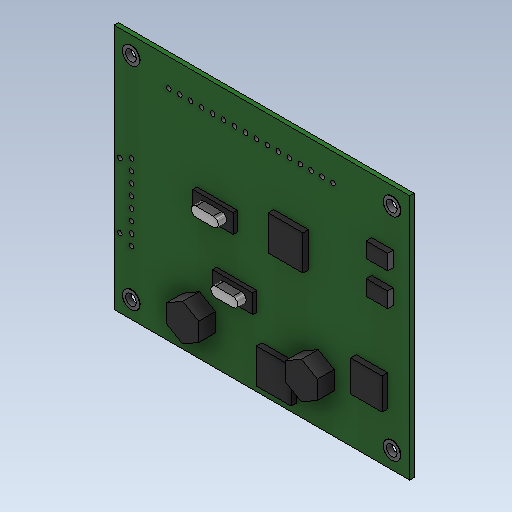
# Autodesk Inventor part: CPU_PCB
Saved by Autodesk Inventor 2020.1 (Build 241239000, 239)
## iProperties
Created: 2005-03-02
Part Number: CPU_PCB
Document SubType Name: Modeling
Designer: Autodesk
Density: 1 g/cm^3
Mass: 20.0863 g
Surface Area: 248.892 cm^2
Volume: 20.0863 cm^3
Material: Generic
Appearance: Default
Total Footprint: 0.000 kg
Author: Autodesk
Autodesk Inventor part; units mm, degrees
ref_plane "YZ Plane" through (0, 0, 0) normal (1, 0, 0) x (0, 1, 0)
ref_plane "XZ Plane" through (0, 0, 0) normal (0, 1, 0) x (-1, 0, 0)
ref_plane "XY Plane" through (0, 0, 0) normal (0, 0, 1) x (1, 0, 0)
sketch "Sketch1" plane through (0, 0, 0) normal (0, 0, 1) x (1, 0, 0)
  line L0 (-6.35, -62.4) -> (101.65, -62.4)
  line L1 (101.65, -62.4) -> (101.65, -152.4)
  line L2 (101.65, -152.4) -> (-6.35, -152.4)
  line L3 (-6.35, -152.4) -> (-6.35, -62.4)
  line L4 (0, -68.75) -> (95.3, -68.75) construction
  line L5 (95.3, -68.75) -> (95.3, -146.05) construction
  line L6 (95.3, -146.05) -> (0, -146.05) construction
  line L7 (0, -146.05) -> (0, -68.75) construction
  circle A0 centre (0, -146.05) radius 1.9812
  circle A1 centre (95.3, -146.05) radius 1.9812
  circle A2 centre (95.3, -68.75) radius 1.9812
  circle A3 centre (0, -68.75) radius 1.9812
  point P0 (47.65, -152.4)
  point P1 (47.65, -146.05)
  point P2 (-6.35, -107.4)
  point P3 (0, -107.4)
  dimension "d0" = 6.35
  dimension "d1" = 6.35
  dimension "d2" = 3.9624
  dimension "d84" = 90
  dimension "d85" = 108
  constraints: 16 end point, 4 centre point, 4 coincident, 4 midpoint, 4 parallel, 3 equal radius, 2 horizontal, 2 perpendicular, 1 horizontal alignment, 1 vertical alignment, 1 other
  measures "d0" distance between parallel lines of L3 L7
  measures "d1" distance between parallel lines of L0 L4
  measures "d2" diameter of A0
  measures "d84" distance between parallel lines of L2 L0
  measures "d85" distance between parallel lines of L3 L1
extrude "Extrusion1" add sketch "Sketch1" along normal blind 1.5875
sketch "Sketch2" plane through (0, 0, 1.5875) normal (0, 0, 1) x (1, 0, 0)
  circle A0 centre (0, -68.75) radius 1.9812 projected
  circle A1 centre (95.3, -68.75) radius 1.9812 projected
  circle A2 centre (95.3, -146.05) radius 1.9812 projected
  circle A3 centre (0, -146.05) radius 1.9812 projected
  line L0 (101.65, -62.4) -> (101.65, -152.4) projected
  line L1 (-6.35, -62.4) -> (101.65, -62.4) projected
  line L2 (-6.35, -152.4) -> (-6.35, -62.4) projected
  line L3 (101.65, -152.4) -> (-6.35, -152.4) projected
  circle A4 centre (0, -68.75) radius 3.175
  circle A5 centre (95.3, -68.75) radius 3.175
  circle A6 centre (95.3, -146.05) radius 3.175
  circle A7 centre (0, -146.05) radius 3.175
  dimension "d5" = 6.35
  constraints: 4 centre point, 4 coincident, 3 equal radius
  measures "d5" diameter of A7
extrude "Extrusion2" add sketch "Sketch2" along normal blind 0.1984 contours A4 | A5 | A6 | A7
sketch "Sketch3" plane through (0, 0, 0) normal (0, 0, -1) x (-1, 0, 0)
  circle A0 centre (0, -68.75) radius 1.9812 projected
  circle A1 centre (-95.3, -68.75) radius 1.9812 projected
  circle A2 centre (-95.3, -146.05) radius 1.9812 projected
  circle A3 centre (0, -146.05) radius 1.9812 projected
  line L0 (6.35, -62.4) -> (-101.65, -62.4) projected
  line L1 (-101.65, -62.4) -> (-101.65, -152.4) projected
  line L2 (-101.65, -152.4) -> (6.35, -152.4) projected
  line L3 (6.35, -152.4) -> (6.35, -62.4) projected
  circle A4 centre (0, -68.75) radius 3.175
  circle A5 centre (-95.3, -68.75) radius 3.175
  circle A6 centre (-95.3, -146.05) radius 3.175
  circle A7 centre (0, -146.05) radius 3.175
  dimension "d8" = 6.35
  constraints: 4 centre point, 4 coincident, 3 equal radius
  measures "d8" diameter of A4
extrude "Extrusion3" add sketch "Sketch3" along normal blind 0.1984 contours A4 | A5 | A6 | A7
sketch "Sketch4" plane through (0, 0, 1.5875) normal (0, 0, 1) x (1, 0, 0)
  circle A0 centre (95.3, -146.05) radius 3.175 projected
  circle A1 centre (0, -68.75) radius 3.175 projected
  circle A2 centre (95.3, -68.75) radius 3.175 projected
  circle A3 centre (0, -146.05) radius 3.175 projected
  line L0 (101.65, -62.4) -> (101.65, -152.4) projected
  line L1 (-6.35, -62.4) -> (101.65, -62.4) projected
  line L2 (-6.35, -152.4) -> (-6.35, -62.4) projected
  line L3 (101.65, -152.4) -> (-6.35, -152.4) projected
  circle A4 centre (0, -101.4) radius 1.6433
  circle A5 centre (0, -105.3624) radius 1.6433
  circle A6 centre (0, -109.3248) radius 1.6433
  circle A7 centre (0, -113.2872) radius 1.6433
  circle A8 centre (0, -117.2496) radius 1.6433
  circle A9 centre (0, -121.212) radius 1.6433
  circle A10 centre (0, -125.1744) radius 1.6433
  circle A11 centre (0, -129.1368) radius 1.6433
  circle A12 centre (-4.2418, -103.3812) radius 1.6433
  circle A13 centre (-4.2418, -127.1556) radius 1.6433
  line L4 (-6.35, -62.4) -> (101.65, -62.4) projected
  point P0 (13.65, -72.4)
  point P1 (17.65, -72.4)
  point P2 (21.65, -72.4)
  point P3 (25.65, -72.4)
  point P4 (29.65, -72.4)
  point P5 (33.65, -72.4)
  point P6 (37.65, -72.4)
  point P7 (41.65, -72.4)
  point P8 (45.65, -72.4)
  point P9 (49.65, -72.4)
  point P10 (53.65, -72.4)
  point P11 (57.65, -72.4)
  point P12 (61.65, -72.4)
  point P13 (65.65, -72.4)
  point P14 (69.65, -72.4)
  point P15 (73.65, -72.4)
  dimension "d22" = 3.9624
  dimension "d27" = 4.2418
  dimension "d28" = 1.9812
  dimension "d29" = 1.9812
  dimension "d30" = 4.2418
  dimension "d75" = 6.35
  dimension "d76" = 51
  dimension "d79" = 4
  dimension "d86" = 10
  dimension "d87" = 20
  constraints: 10 centre point, 2 equal radius, 1 horizontal, 1 vertical, 29 other
  measures "d22" distance of A4.centre A5.centre
  measures "d27" horizontal distance of A4.centre A12.centre
  measures "d28" vertical distance of A12.centre A4.centre
  measures "d29" vertical distance of A13.centre A11.centre
  measures "d30" horizontal distance of A13.centre A11.centre
  measures "d75" distance from line of L2 A4.centre
  measures "d76" distance from line of A4.centre L3
  measures "d79" distance of point (13.65, -72.4) point (17.65, -72.4)
  measures "d86" distance from line of L1 point (13.65, -72.4)
  measures "d87" distance from line of L2 point (13.65, -72.4)
hole "Hole1" at (13.65, -72.4, 1.5875) at (0, -101.4, 1.5875) at (0, -105.3624, 1.5875) at (0, -109.3248, 1.5875) at (0, -113.2872, 1.5875) at (0, -117.2496, 1.5875) at (0, -121.212, 1.5875) at (0, -125.1744, 1.5875) at (0, -129.1368, 1.5875) at (-4.2418, -127.1556, 1.5875) at (-4.2418, -103.3812, 1.5875) at (73.65, -72.4, 1.5875) at (69.65, -72.4, 1.5875) at (65.65, -72.4, 1.5875) at (61.65, -72.4, 1.5875) at (57.65, -72.4, 1.5875) at (53.65, -72.4, 1.5875) at (49.65, -72.4, 1.5875) at (45.65, -72.4, 1.5875) at (37.65, -72.4, 1.5875) at (33.65, -72.4, 1.5875) at (29.65, -72.4, 1.5875) at (25.65, -72.4, 1.5875) at (21.65, -72.4, 1.5875) at (17.65, -72.4, 1.5875) at (41.65, -72.4, 1.5875) direction (0, 0, -1) diameter 1.7018 end through all
sketch "Sketch5" plane through (0, 0, 1.5875) normal (0, 0, 1) x (1, 0, 0)
  line L0 (51.9916, -91.6366) -> (64.6916, -91.6366)
  line L1 (64.6916, -91.6366) -> (64.6916, -104.3366)
  line L2 (64.6916, -104.3366) -> (51.9916, -104.3366)
  line L3 (51.9916, -104.3366) -> (51.9916, -91.6366)
  line L4 (30.3358, -18.3269) -> (55.7358, -18.3269)
  line L5 (55.7358, -18.3269) -> (55.7358, -43.7269)
  line L6 (55.7358, -43.7269) -> (30.3358, -43.7269)
  line L7 (30.3358, -43.7269) -> (30.3358, -18.3269)
  line L8 (47.6872, -135.9105) -> (60.3872, -135.9105)
  line L9 (60.3872, -135.9105) -> (60.3872, -148.6105)
  line L10 (60.3872, -148.6105) -> (47.6872, -148.6105)
  line L11 (47.6872, -148.6105) -> (47.6872, -135.9105)
  line L12 (82.1409, -122.4624) -> (93.5709, -122.4624)
  line L13 (93.5709, -122.4624) -> (93.5709, -133.8924)
  line L14 (93.5709, -133.8924) -> (82.1409, -133.8924)
  line L15 (82.1409, -133.8924) -> (82.1409, -122.4624)
  line L16 (87.7634, -29.3007) -> (95.6374, -29.3007)
  line L17 (95.6374, -29.3007) -> (95.6374, -34.8887)
  line L18 (95.6374, -34.8887) -> (87.7634, -34.8887)
  line L19 (87.7634, -34.8887) -> (87.7634, -29.3007)
  line L20 (87.7634, -41.2387) -> (95.6374, -41.2387)
  line L21 (95.6374, -41.2387) -> (95.6374, -46.8267)
  line L22 (95.6374, -46.8267) -> (87.7634, -46.8267)
  line L23 (87.7634, -46.8267) -> (87.7634, -41.2387)
  line L24 (87.7634, -82.6142) -> (95.6374, -82.6142)
  line L25 (95.6374, -82.6142) -> (95.6374, -88.2022)
  line L26 (95.6374, -88.2022) -> (87.7634, -88.2022)
  line L27 (87.7634, -88.2022) -> (87.7634, -82.6142)
  line L28 (87.7634, -94.5522) -> (95.6374, -94.5522)
  line L29 (95.6374, -94.5522) -> (95.6374, -100.1402)
  line L30 (95.6374, -100.1402) -> (87.7634, -100.1402)
  line L31 (87.7634, -100.1402) -> (87.7634, -94.5522)
  dimension "d38" = 25.4
  dimension "d39" = 25.4
  dimension "d40" = 12.7
  dimension "d41" = 12.7
  dimension "d42" = 12.7
  dimension "d43" = 12.7
  dimension "d44" = 11.43
  dimension "d45" = 11.43
  dimension "d48" = 7.874
  dimension "d49" = 5.588
  dimension "d50" = 6.35
  dimension "d51" = 35.7875
  dimension "d52" = 6.35
  constraints: 64 end point, 16 parallel, 8 horizontal, 8 perpendicular, 6 equal length, 3 vertical alignment
  measures "d38" distance of L4.start L4.end
  measures "d39" distance of L6.end L4.start
  measures "d40" distance of L1.end L2.end
  measures "d41" distance of L2.end L0.start
  measures "d42" distance of L9.end L10.end
  measures "d43" distance of L8.end L9.end
  measures "d44" distance of L14.end L12.start
  measures "d45" distance of L13.end L14.end
  measures "d48" distance of L16.start L16.end
  measures "d49" distance of L18.end L16.start
  measures "d50" distance between parallel lines of L20 L18
  measures "d51" distance between parallel lines of L24 L22
  measures "d52" distance between parallel lines of L28 L26
extrude "Extrusion4" add sketch "Sketch5" along normal blind 2.032 contours L0 L1 L2 L3 | L8 L9 L10 L11 | L12 L13 L14 L15 | L24 L25 L26 L27 | L28 L29 L30 L31
sketch "Sketch6" plane through (0, 0, 1.5875) normal (0, 0, 1) x (1, 0, 0)
  line L0 (23.9571, -98.5044) -> (38.6891, -98.5044)
  line L1 (38.6891, -98.5044) -> (38.6891, -105.3624)
  line L2 (38.6891, -105.3624) -> (23.9571, -105.3624)
  line L3 (23.9571, -105.3624) -> (23.9571, -98.5044)
  line L4 (31.107, -120.3013) -> (45.839, -120.3013)
  line L5 (45.839, -120.3013) -> (45.839, -127.1593)
  line L6 (45.839, -127.1593) -> (31.107, -127.1593)
  line L7 (31.107, -127.1593) -> (31.107, -120.3013)
  dimension "d53" = 6.858
  dimension "d54" = 14.732
  dimension "d55" = 6.858
  dimension "d56" = 14.732
  constraints: 16 end point, 4 parallel, 2 horizontal, 2 perpendicular
  measures "d53" distance of L0.end L1.end
  measures "d54" distance of L1.end L2.end
  measures "d55" distance of L4.end L5.end
  measures "d56" distance of L5.end L6.end
extrude "Extrusion5" add sketch "Sketch6" along normal blind 1.524
sketch "Sketch7" plane through (0, 0, 3.1115) normal (0, 0, 1) x (1, 0, 0)
  line L0 (23.9571, -98.5044) -> (38.6891, -98.5044) projected
  line L1 (23.9571, -105.3624) -> (23.9571, -98.5044) projected
  arc A0 (28.1751, -100.1556) -> (28.2466, -103.7087) centre (28.1481, -101.9334) ccw
  arc A1 (34.3961, -103.7085) -> (34.4981, -100.1554) centre (34.4981, -101.9334) ccw
  arc A2 (35.3184, -121.9524) -> (35.3085, -125.5083) centre (35.298, -123.7303) ccw
  arc A3 (41.648, -125.5083) -> (41.6479, -121.9523) centre (41.648, -123.7303) ccw
  line L2 (45.839, -120.3013) -> (45.839, -127.1593) projected
  line L3 (31.107, -120.3013) -> (45.839, -120.3013) projected
  line L4 (31.107, -127.1593) -> (31.107, -120.3013) projected
  line L5 (45.839, -127.1593) -> (31.107, -127.1593) projected
  line L6 (28.1481, -101.9334) -> (34.4981, -101.9334) construction
  line L7 (28.121, -100.1556) -> (34.4981, -100.1554)
  line L8 (28.0498, -103.7087) -> (34.6002, -103.7085)
  line L9 (35.298, -123.7303) -> (41.648, -123.7303) construction
  line L10 (31.107, -127.1593) -> (31.107, -120.3013) projected
  line L11 (35.2774, -121.9524) -> (41.6479, -121.9523)
  line L12 (35.2874, -125.5083) -> (41.648, -125.5083)
  point P0 (31.3231, -101.9334)
  point P1 (31.3231, -98.5044)
  point P2 (23.9571, -101.9334)
  point P3 (38.473, -123.7303)
  point P4 (31.107, -123.7303)
  point P5 (38.473, -120.3013)
  point P6 (31.107, -123.7303)
  point P7 (31.107, -123.7303)
  dimension "d59" = 3.556
  dimension "d60" = 6.35
  dimension "d61" = 6.35
  constraints: 13 point on circle, 12 end point, 8 midpoint, 5 horizontal alignment, 5 point on line, 4 centre point, 3 equal radius, 3 tangent, 2 vertical alignment, 1 parallel
  measures "d59" diameter of A0
  measures "d60" distance of L6.end L6.start
  measures "d61" distance of L9.start L9.end
extrude "Extrusion6" add sketch "Sketch7" along normal blind 3.048 contours L7 A1 L8 A0 | L11 A3 L12 A2
sketch "Sketch8" plane through (0, 0, 1.5875) normal (0, 0, 1) x (1, 0, 0)
  line L0 (101.65, -62.4) -> (101.65, -152.4) projected
  line L1 (68.2146, -141.3088) -> (62.3726, -137.9359)
  line L2 (62.3726, -137.9359) -> (62.3726, -131.1902)
  line L3 (62.3726, -131.1902) -> (68.2146, -127.8173)
  line L4 (68.2146, -127.8173) -> (74.0566, -131.1902)
  line L5 (74.0566, -131.1902) -> (74.0566, -137.9359)
  line L6 (74.0566, -137.9359) -> (68.2146, -141.3088)
  line L7 (24.808, -144.6817) -> (18.966, -141.3088)
  line L8 (18.966, -141.3088) -> (18.966, -134.5631)
  line L9 (18.966, -134.5631) -> (24.808, -131.1902)
  line L10 (24.808, -131.1902) -> (30.65, -134.5631)
  line L11 (30.65, -134.5631) -> (30.65, -141.3088)
  line L12 (30.65, -141.3088) -> (24.808, -144.6817)
  point P0 (68.2146, -134.5631)
  point P1 (24.808, -137.9359)
  dimension "d64" = 11.684
  dimension "d65" = 11.684
  constraints: 24 end point, 2 parallel, 22 other
  measures "d64" distance between parallel lines of L6 L3
  measures "d65" distance between parallel lines of L12 L9
extrude "Extrusion7" add sketch "Sketch8" along normal blind 6.096
body "Solid1"
